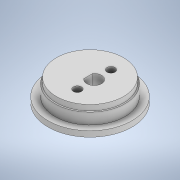
# Autodesk Inventor part: Rotor_shaft_21
Saved by Autodesk Inventor 2021 (Build 250183000, 183)
## iProperties
Created: 2022-08-07
Part Number: Rotor_shaft_21
Material: Ogólny
Document SubType Name: Modeling
Designer: MicnedSQ
Density: 1 g/cm^3
Appearance: Domyślna
Author: MicnedSQ
Autodesk Inventor part; units mm, degrees
ref_plane "YZ Plane" through (0, 0, 0) normal (1, 0, 0) x (0, 1, 0)
ref_plane "XZ Plane" through (0, 0, 0) normal (0, 1, 0) x (-1, 0, 0)
ref_plane "XY Plane" through (0, 0, 0) normal (0, 0, 1) x (1, 0, 0)
sketch "Szkic1" plane through (0, 0, 0) normal (0, 1, 0) x (-1, 0, 0)
  circle A0 centre (0, 0) radius 15
  dimension "d0" = 30
  constraints: 1 centre point, 1 coincident
  measures "d0" diameter of A0
extrude "Wyciągnięcie proste1" add sketch "Szkic1" along normal blind 2
sketch "Szkic2" plane through (0, 2, 0) normal (0, 1, 0) x (1, 0, 0)
  circle A0 centre (0, 0) radius 12.5
  dimension "d3" = 25
  constraints: 1 centre point, 1 coincident
  measures "d3" diameter of A0
extrude "Wyciągnięcie proste2" add sketch "Szkic2" along normal blind 4
sketch "Szkic9" plane through (0, 6, 0) normal (0, 1, 0) x (1, 0, 0)
  circle A0 centre (0, 0) radius 12
  dimension "d22" = 24
  constraints: 1 centre point, 1 coincident
  measures "d22" diameter of A0
extrude "Wyciągnięcie proste7" add sketch "Szkic9" along normal blind 2
sketch "Szkic11" plane through (0, 8, 0) normal (0, 1, 0) x (1, 0, 0)
  circle A0 centre (1.5, -6) radius 1.45
  circle A1 centre (1.5, 6) radius 1.45
  point P0 (0, 0)
  dimension "d25" = 2.9
  dimension "d26" = 2.9
  constraints: 2 centre point, 2 coincident
  measures "d25" diameter of A0
  measures "d26" diameter of A1
extrude "Wyciągnięcie proste8" cut sketch "Szkic11" against normal blind 6
sketch "Szkic5" plane through (0, 0, 0) normal (0, -1, 0) x (1, 0, 0)
  arc A0 (-0.62, -1.59) -> (-0.62, 1.59) centre (1.5, 0) ccw
  line L0 (-0.62, 1.59) -> (-0.62, -1.59)
  point P0 (0, 0)
  constraints: 2 end point, 2 point on circle, 1 centre point, 1 vertical
extrude "Wyciągnięcie proste5" cut sketch "Szkic5" against normal blind 8
